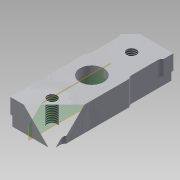
# Autodesk Inventor part: Part25
Saved by Autodesk Inventor 2016 (Build 200138000, 138)
## iProperties
Created: 2016-01-20
Part Number: Part25
Material: PAEK Plastic
Document SubType Name: Modeling
Designer: admin
Density: 1.32 g/cm^3
Appearance: Smooth - White
Mass: 2.05469 g
Surface Area: 14.0166 cm^2
Volume: 1.55658 cm^3
Author: admin
Autodesk Inventor part; units mm, degrees
ref_plane "YZ Plane" through (0, 0, 0) normal (1, 0, 0) x (0, 1, 0)
ref_plane "XZ Plane" through (0, 0, 0) normal (0, 1, 0) x (-1, 0, 0)
ref_plane "XY Plane" through (0, 0, 0) normal (0, 0, 1) x (1, 0, 0)
sketch "Sketch1" plane through (0, 0, 0) normal (0, 0, 1) x (1, 0, 0)
  line L0 (-5.5, -15) -> (5.5, -15)
  line L1 (5.5, -15) -> (5.5, 15)
  line L2 (5.5, 15) -> (-5.5, 15)
  line L3 (-5.5, 15) -> (-5.5, -15)
  line L4 (-5.5, -15) -> (5.5, 15) construction
  line L5 (5.5, -15) -> (-5.5, 15) construction
  circle A0 centre (0, 0) radius 3 projected
  circle A1 centre (0, 0) radius 3.7 projected
  dimension "d0" = 5.5
  dimension "d1" = 15
  constraints: 12 end point, 2 parallel, 1 horizontal, 1 perpendicular
  measures "d0" distance from line of L1 point (0, 0)
  measures "d1" distance from line of L2 point (0, 0)
extrude "Extrusion1" add sketch "Sketch1" along normal blind 2 contours L3 L2 L1 L0 | A0 | A1
sketch "Sketch2" plane through (0, 0, 0) normal (0, 0, -1) x (-1, 0, 0)
  line L0 (5.5, -15) -> (-5.5, -15) projected
  line L1 (5.5, 15) -> (5.5, -15) projected
  line L2 (-5.5, 15) -> (5.5, 15) projected
  line L3 (-5.5, -15) -> (-5.5, 15) projected
  circle A0 centre (0, 0) radius 4 projected
extrude "Extrusion2" add sketch "Sketch2" along normal blind 4
sketch "Sketch3" plane through (0, 0, 2) normal (0, 0, 1) x (1, 0, 0)
  line L0 (-5.5, -15) -> (5.5, -15) projected
  line L1 (5.5, 15) -> (-5.5, 15) projected
  circle A0 centre (0, 10) radius 1.2
  circle A1 centre (0, -10) radius 1.2
  dimension "d6" = 2.4
  dimension "d7" = 2.4
  dimension "d8" = 5
  dimension "d9" = 5
  constraints: 2 centre point
  measures "d6" diameter of A0
  measures "d7" diameter of A1
  measures "d8" distance from line of L0 A1.centre
  measures "d9" distance from line of L1 A0.centre
extrude "Extrusion3" cut sketch "Sketch3" against normal blind 10
sketch "Sketch6" plane through (0, 0, -4) normal (0, 0, -1) x (-1, 0, 0)
  line L0 (-5.5, -15) -> (5.5, -15) projected
  line L1 (5.5, -15) -> (5.5, 15) projected
  line L2 (-5.5, 15) -> (-5.5, -15) projected
  line L3 (5.5, 12) -> (5.5, 13.2929) projected
  line L4 (5.5, -15) -> (5.5, -13.7071) projected
  line L5 (5.5, 12) -> (-5.5, 12)
  arc A0 (5, 5) -> (5.5, 3.882) centre (6.5, 5) ccw
  line L6 (5, 11.5) -> (5, 5)
  arc A1 (5.5, -12.3842) -> (5, -13.7071) centre (7, -13.7071) ccw
  line L7 (5, -13.7071) -> (5, -15)
  arc A2 (5.5, 12.618) -> (5, 11.5) centre (6.5, 11.5) ccw
  line L8 (5.5, 15) -> (-5.5, 15) projected
  dimension "d23" = 3
  dimension "d25" = 4
  dimension "d38" = 10
  dimension "d39" = 3.5
  dimension "d40" = 0.5
  dimension "d41" = 1.5
  constraints: 6 end point, 6 point on circle, 5 point on line, 3 centre point, 3 tangent, 1 collinear, 1 perpendicular
  measures "d23" diameter of A0
  measures "d25" diameter of A1
  measures "d38" distance from line of L8 A0.centre
  measures "d39" distance from line of L8 A2.centre
  measures "d40" distance between parallel lines of L1 L6
  measures "d41" radius of A2
sketch "Sketch7" plane through (0, 0, -4) normal (0, 0, -1) x (-1, 0, 0)
  arc A0 (5.5, 12.8229) -> (5, 11.5) centre (7, 11.5) ccw projected
  line L0 (5.5, 15) -> (-5.5, 15) projected
  line L1 (-5.5, -15) -> (5.5, -15) projected
  line L2 (5.5, -15) -> (5.5, 15) projected
  line L3 (5, 5) -> (5, 11.5) projected
  line L4 (5, 11.5) -> (5, 15)
  arc A1 (5.5, -11.882) -> (5, -13) centre (6.5, -13) ccw
  line L5 (5, -13) -> (5, -15)
  line L6 (5, -15) -> (5.5, -15)
  line L7 (5.5, -15) -> (5.5, -11.882)
  line L8 (5.5, -15) -> (5.5, 15) projected
  line L9 (5, 15) -> (5.5, 15)
  line L10 (5.5, 15) -> (5.5, 12.8229)
  line L11 (5.5, 12.8229) -> (5.5, 11.5)
  line L12 (5.5, 11.5) -> (5.5, 10.597)
  line L13 (5.5, 10.597) -> (5, 10.597)
  line L14 (5, 10.597) -> (5, 11.5)
  point P0 (5.5, 3.6771)
  dimension "d29" = 3
  dimension "d30" = 2
  dimension "d51" = 0.5
  constraints: 20 end point, 5 collinear, 3 point on line, 2 point on circle, 2 tangent, 1 centre point, 1 parallel, 1 perpendicular
  measures "d29" diameter of A1
  measures "d30" distance from line of L1 A1.centre
  measures "d51" distance between parallel lines of L2 L5
extrude "Extrusion8" cut sketch "Sketch6" against normal blind 100 contours A2 L1 L5 | L5 L1 A0 L6 A2
extrude "Extrusion9" cut sketch "Sketch7" against normal blind 2.2
ref_plane "Work Plane1" through (0, -15, 2) normal (-1, 0, 0) x (0, 0, 1)
mirror "Mirror1" about plane through (0, -15, 2) normal (-1, 0, 0) of "Extrusion9", "Extrusion8"
sketch "Sketch8" plane through (0, 0, -4) normal (0, 0, -1) x (-1, 0, 0)
  circle A0 centre (0, 10) radius 1.2 projected
  circle A1 centre (0, -10) radius 1.2 projected
  circle A2 centre (0, 0) radius 4 projected
  line L0 (-5, 15) -> (-5, 5) projected
  arc A3 (-5.5, 3.882) -> (-5, 5) centre (-6.5, 5) ccw projected
  line L1 (-5.5, 3.882) -> (-5.5, -11.882) projected
  arc A4 (-5, -13) -> (-5.5, -11.882) centre (-6.5, -13) ccw projected
  line L2 (-5, -13) -> (-5, -15) projected
  line L3 (-5, -15) -> (5, -15) projected
  line L4 (5, -15) -> (5, -13) projected
  arc A5 (5.5, -11.882) -> (5, -13) centre (6.5, -13) ccw projected
  line L5 (5.5, -11.882) -> (5.5, 3.882) projected
  arc A6 (5, 5) -> (5.5, 3.882) centre (6.5, 5) ccw projected
  line L6 (5, 5) -> (5, 15) projected
  line L7 (5, 15) -> (-5, 15) projected
extrude "Extrusion10" add sketch "Sketch8" along normal blind 0.2
sketch "Sketch9" plane through (0, 0, 0) normal (0, 0, -1) x (-1, 0, 0)
  circle A0 centre (0, 0) radius 4 projected
  circle A1 centre (0, 0) radius 3
  dimension "d44" = 6
  constraints: 1 centre point, 1 coincident
  measures "d44" diameter of A1
extrude "Extrusion11" cut sketch "Sketch9" against normal blind 100 contours A1
thread "Thread1" size "M3x0.5" class "6H" standard "ANSI Metric M Profile" full length
thread "Thread2" size "M3x0.5" class "6H" standard "ANSI Metric M Profile" full length
body "Solid1"
